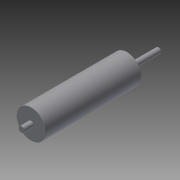
# Autodesk Inventor part: Conveyor Axle
Saved by Autodesk Inventor 2015 (Build 190159000, 159)
## iProperties
Created: 2015-01-11
Part Number: Conveyor Axle
Material: Generic
Document SubType Name: Modeling
Designer: chapale16
Density: 1 g/cm^3
Appearance: Default
Author: chapale16
Autodesk Inventor part; units mm, degrees
ref_plane "YZ Plane" through (0, 0, 0) normal (1, 0, 0) x (0, 1, 0)
ref_plane "XZ Plane" through (0, 0, 0) normal (0, 1, 0) x (-1, 0, 0)
ref_plane "XY Plane" through (0, 0, 0) normal (0, 0, 1) x (1, 0, 0)
sketch "Sketch1" plane through (0, 0, 0) normal (0, 0, 1) x (1, 0, 0)
  circle A0 centre (0, 0) radius 7.3025
  dimension "d0" = 14.605
  constraints: 1 centre point, 1 coincident
  measures "d0" diameter of A0
extrude "Extrusion1" add sketch "Sketch1" along normal blind 421.005
sketch "Sketch2" plane through (0, 0, 421.005) normal (0, 0, 1) x (1, 0, 0)
  circle A0 centre (0, 0) radius 9.017
  circle A1 centre (0, 0) radius 12.7
  dimension "d3" = 18.034
  dimension "d4" = 25.4
  constraints: 2 centre point, 2 coincident
  measures "d3" diameter of A0
  measures "d4" diameter of A1
extrude "Extrusion2" add sketch "Sketch2" against normal blind 457.2
sketch "Sketch3" plane through (0, 0, 421.005) normal (0, 0, 1) x (1, 0, 0)
  circle A0 centre (0, 0) radius 7.3025
  circle A1 centre (0, 0) radius 12.7
  circle A2 centre (0, 0) radius 8.9258
  constraints: 3 centre point, 3 coincident
extrude "Extrusion3" cut sketch "Sketch3" against normal blind 508 contours A1
sketch "Sketch5" plane through (0, 0, 421.005) normal (0, 0, 1) x (1, 0, 0)
  circle A0 centre (0, 0) radius 38.1
  dimension "d12" = 76.2
  constraints: 1 centre point, 1 coincident
  measures "d12" diameter of A0
extrude "Extrusion5" add sketch "Sketch5" against normal blind 337.5025
sketch "Sketch7" plane through (0, 0, 421.005) normal (0, 0, 1) x (1, 0, 0)
  circle A0 centre (0, 0) radius 7.3768
  circle A1 centre (0, 0) radius 38.1
  constraints: 2 centre point, 2 coincident
extrude "Extrusion6" cut sketch "Sketch7" against normal blind 83.5025
sketch "Sketch9" plane through (0, 0, 421.005) normal (0, 0, 1) x (1, 0, 0)
  circle A0 centre (0, 0) radius 7.3025
  circle A1 centre (0, 0) radius 10.3013
  constraints: 2 centre point, 2 coincident
extrude "Extrusion7" cut sketch "Sketch9" against normal blind 58.1025 contours A0 | A1
body "Solid1"
